Autodesk Fusion 360 part; units mm, degrees
(part 2 of 2)
  arc A37 (11.8839, 4.6211) -> (11.6708, 5.1356) centre (0, 0) ccw
  spline S74 degree 3 poles (11.6708, 5.1356) (11.1523, 5.1719) (10.7664, 5.1326) (10.5094, 5.0835) knots 0 0 0 0 1 1 1 1
  spline S75 degree 3 poles (10.5094, 5.0835) (10.2945, 5.0423) (10.1746, 4.996) (10.1353, 4.9792) knots 0 0 0 0 1 1 1 1
  line L38 (10.1353, 4.9792) -> (9.929, 4.8779)
  arc A38 (9.929, 4.8779) -> (9.5721, 5.5457) centre (0, 0) ccw
  line L39 (9.5721, 5.5457) -> (9.771, 5.6609)
  spline S76 degree 3 poles (9.771, 5.6609) (9.8067, 5.6842) (9.9118, 5.7583) (10.0655, 5.914) knots 0 0 0 0 1 1 1 1
  spline S77 degree 3 poles (10.0655, 5.914) (10.2491, 6.1004) (10.4962, 6.3994) (10.754, 6.8508) knots 0 0 0 0 1 1 1 1
  arc A39 (10.754, 6.8508) -> (10.4447, 7.3137) centre (0, 0) ccw
  spline S78 degree 3 poles (10.4447, 7.3137) (9.929, 7.2483) (9.5582, 7.1344) (9.3157, 7.0361) knots 0 0 0 0 1 1 1 1
  spline S79 degree 3 poles (9.3157, 7.0361) (9.113, 6.9538) (9.0044, 6.8849) (8.9692, 6.8609) knots 0 0 0 0 1 1 1 1
  line L40 (8.9692, 6.8609) -> (8.7866, 6.7212)
  arc A40 (8.7866, 6.7212) -> (8.3062, 7.3065) centre (0, 0) ccw
  line L41 (8.3062, 7.3065) -> (8.4788, 7.4584)
  spline S80 degree 3 poles (8.4788, 7.4584) (8.5093, 7.4882) (8.598, 7.5813) (8.7184, 7.7641) knots 0 0 0 0 1 1 1 1
  spline S81 degree 3 poles (8.7184, 7.7641) (8.862, 7.9827) (9.046, 8.3242) (9.2109, 8.8171) knots 0 0 0 0 1 1 1 1
  arc A41 (9.2109, 8.8171) -> (8.8171, 9.2109) centre (0, 0) ccw
  spline S82 degree 3 poles (8.8171, 9.2109) (8.3242, 9.046) (7.9827, 8.862) (7.7641, 8.7184) knots 0 0 0 0 1 1 1 1
  spline S83 degree 3 poles (7.7641, 8.7184) (7.5813, 8.598) (7.4882, 8.5093) (7.4584, 8.4788) knots 0 0 0 0 1 1 1 1
  line L42 (7.4584, 8.4788) -> (7.3065, 8.3062)
  arc A42 (7.3065, 8.3062) -> (6.7212, 8.7866) centre (0, 0) ccw
  line L43 (6.7212, 8.7866) -> (6.8609, 8.9692)
  spline S84 degree 3 poles (6.8609, 8.9692) (6.8849, 9.0044) (6.9538, 9.113) (7.0361, 9.3157) knots 0 0 0 0 1 1 1 1
  spline S85 degree 3 poles (7.0361, 9.3157) (7.1344, 9.5582) (7.2483, 9.929) (7.3137, 10.4447) knots 0 0 0 0 1 1 1 1
  arc A43 (7.3137, 10.4447) -> (6.8508, 10.754) centre (0, 0) ccw
  spline S86 degree 3 poles (6.8508, 10.754) (6.3994, 10.4962) (6.1004, 10.2491) (5.914, 10.0655) knots 0 0 0 0 1 1 1 1
  spline S87 degree 3 poles (5.914, 10.0655) (5.7583, 9.9118) (5.6842, 9.8067) (5.6609, 9.771) knots 0 0 0 0 1 1 1 1
  line L44 (5.6609, 9.771) -> (5.5457, 9.5721)
  arc A44 (5.5457, 9.5721) -> (4.8779, 9.929) centre (0, 0) ccw
  line L45 (4.8779, 9.929) -> (4.9792, 10.1353)
  spline S88 degree 3 poles (4.9792, 10.1353) (4.996, 10.1746) (5.0423, 10.2945) (5.0835, 10.5094) knots 0 0 0 0 1 1 1 1
  spline S89 degree 3 poles (5.0835, 10.5094) (5.1326, 10.7664) (5.1719, 11.1523) (5.1356, 11.6708) knots 0 0 0 0 1 1 1 1
  arc A45 (5.1356, 11.6708) -> (4.6211, 11.8839) centre (0, 0) ccw
  spline S90 degree 3 poles (4.6211, 11.8839) (4.2287, 11.543) (3.9837, 11.2423) (3.8367, 11.0259) knots 0 0 0 0 1 1 1 1
  spline S91 degree 3 poles (3.8367, 11.0259) (3.7139, 10.8448) (3.6618, 10.7272) (3.6459, 10.6876) knots 0 0 0 0 1 1 1 1
  line L46 (3.6459, 10.6876) -> (3.5717, 10.47)
  arc A46 (3.5717, 10.47) -> (2.8471, 10.6899) centre (0, 0) ccw
  line L47 (2.8471, 10.6899) -> (2.9063, 10.912)
  spline S92 degree 3 poles (2.9063, 10.912) (2.915, 10.9537) (2.937, 11.0804) (2.9356, 11.2992) knots 0 0 0 0 1 1 1 1
  spline S93 degree 3 poles (2.9356, 11.2992) (2.9336, 11.5608) (2.8969, 11.947) (2.76, 12.4485) knots 0 0 0 0 1 1 1 1
  arc A47 (2.76, 12.4485) -> (2.2139, 12.5571) centre (0, 0) ccw
  spline S94 degree 3 poles (2.2139, 12.5571) (1.8956, 12.1462) (1.7139, 11.8034) (1.6119, 11.5625) knots 0 0 0 0 1 1 1 1
  spline S95 degree 3 poles (1.6119, 11.5625) (1.5268, 11.3609) (1.4987, 11.2354) (1.4908, 11.1935) knots 0 0 0 0 1 1 1 1
  line L48 (1.4908, 11.1935) -> (1.4605, 10.9657)
  arc A48 (1.4605, 10.9657) -> (0.7069, 11.0399) centre (0, 0) ccw
  line L49 (0.7069, 11.0399) -> (0.7216, 11.2693)
  spline S96 degree 3 poles (0.7216, 11.2693) (0.7221, 11.3119) (0.7189, 11.4405) (0.6748, 11.6548) knots 0 0 0 0 1 1 1 1
  spline S97 degree 3 poles (0.6748, 11.6548) (0.6218, 11.911) (0.5105, 12.2826) (0.2784, 12.7477) knots 0 0 0 0 1 1 1 1
  arc A49 (0.2784, 12.7477) -> (-0.2784, 12.7477) centre (0, 0) ccw
  spline S98 degree 3 poles (-0.2784, 12.7477) (-0.5105, 12.2826) (-0.6218, 11.911) (-0.6748, 11.6548) knots 0 0 0 0 1 1 1 1
  spline S99 degree 3 poles (-0.6748, 11.6548) (-0.7189, 11.4405) (-0.7221, 11.3119) (-0.7216, 11.2693) knots 0 0 0 0 1 1 1 1
  line L50 (-0.7216, 11.2693) -> (-0.7069, 11.0399)
  arc A50 (-0.7069, 11.0399) -> (-1.4605, 10.9657) centre (0, 0) ccw
  line L51 (-1.4605, 10.9657) -> (-1.4908, 11.1935)
  spline S100 degree 3 poles (-1.4908, 11.1935) (-1.4987, 11.2354) (-1.5268, 11.3609) (-1.6119, 11.5625) knots 0 0 0 0 1 1 1 1
  spline S101 degree 3 poles (-1.6119, 11.5625) (-1.7139, 11.8034) (-1.8956, 12.1462) (-2.2139, 12.5571) knots 0 0 0 0 1 1 1 1
  arc A51 (-2.2139, 12.5571) -> (-2.76, 12.4485) centre (0, 0) ccw
  spline S102 degree 3 poles (-2.76, 12.4485) (-2.8969, 11.947) (-2.9336, 11.5608) (-2.9356, 11.2992) knots 0 0 0 0 1 1 1 1
  spline S103 degree 3 poles (-2.9356, 11.2992) (-2.937, 11.0804) (-2.915, 10.9537) (-2.9063, 10.912) knots 0 0 0 0 1 1 1 1
  line L52 (-2.9063, 10.912) -> (-2.8471, 10.6899)
  arc A52 (-2.8471, 10.6899) -> (-3.5717, 10.47) centre (0, 0) ccw
  line L53 (-3.5717, 10.47) -> (-3.6459, 10.6876)
  spline S104 degree 3 poles (-3.6459, 10.6876) (-3.6618, 10.7272) (-3.7139, 10.8448) (-3.8367, 11.0259) knots 0 0 0 0 1 1 1 1
  spline S105 degree 3 poles (-3.8367, 11.0259) (-3.9837, 11.2423) (-4.2287, 11.543) (-4.6211, 11.8839) knots 0 0 0 0 1 1 1 1
  arc A53 (-4.6211, 11.8839) -> (-5.1356, 11.6708) centre (0, 0) ccw
  spline S106 degree 3 poles (-5.1356, 11.6708) (-5.1719, 11.1523) (-5.1326, 10.7664) (-5.0835, 10.5094) knots 0 0 0 0 1 1 1 1
  spline S107 degree 3 poles (-5.0835, 10.5094) (-5.0423, 10.2945) (-4.996, 10.1746) (-4.9792, 10.1353) knots 0 0 0 0 1 1 1 1
  line L54 (-4.9792, 10.1353) -> (-4.8779, 9.929)
  arc A54 (-4.8779, 9.929) -> (-5.5457, 9.5721) centre (0, 0) ccw
  line L55 (-5.5457, 9.5721) -> (-5.6609, 9.771)
  spline S108 degree 3 poles (-5.6609, 9.771) (-5.6842, 9.8067) (-5.7583, 9.9118) (-5.914, 10.0655) knots 0 0 0 0 1 1 1 1
  spline S109 degree 3 poles (-5.914, 10.0655) (-6.1004, 10.2491) (-6.3994, 10.4962) (-6.8508, 10.754) knots 0 0 0 0 1 1 1 1
  arc A55 (-6.8508, 10.754) -> (-7.3137, 10.4447) centre (0, 0) ccw
  spline S110 degree 3 poles (-7.3137, 10.4447) (-7.2483, 9.929) (-7.1344, 9.5582) (-7.0361, 9.3157) knots 0 0 0 0 1 1 1 1
  spline S111 degree 3 poles (-7.0361, 9.3157) (-6.9538, 9.113) (-6.8849, 9.0044) (-6.8609, 8.9692) knots 0 0 0 0 1 1 1 1
  line L56 (-6.8609, 8.9692) -> (-6.7212, 8.7866)
  arc A56 (-6.7212, 8.7866) -> (-7.3065, 8.3062) centre (0, 0) ccw
  line L57 (-7.3065, 8.3062) -> (-7.4584, 8.4788)
  spline S112 degree 3 poles (-7.4584, 8.4788) (-7.4882, 8.5093) (-7.5813, 8.598) (-7.7641, 8.7184) knots 0 0 0 0 1 1 1 1
  spline S113 degree 3 poles (-7.7641, 8.7184) (-7.9827, 8.862) (-8.3242, 9.046) (-8.8171, 9.2109) knots 0 0 0 0 1 1 1 1
  arc A57 (-8.8171, 9.2109) -> (-9.2109, 8.8171) centre (0, 0) ccw
  spline S114 degree 3 poles (-9.2109, 8.8171) (-9.046, 8.3242) (-8.862, 7.9827) (-8.7184, 7.7641) knots 0 0 0 0 1 1 1 1
  spline S115 degree 3 poles (-8.7184, 7.7641) (-8.598, 7.5813) (-8.5093, 7.4882) (-8.4788, 7.4584) knots 0 0 0 0 1 1 1 1
  line L58 (-8.4788, 7.4584) -> (-8.3062, 7.3065)
  arc A58 (-8.3062, 7.3065) -> (-8.7866, 6.7212) centre (0, 0) ccw
  line L59 (-8.7866, 6.7212) -> (-8.9692, 6.8609)
  spline S116 degree 3 poles (-8.9692, 6.8609) (-9.0044, 6.8849) (-9.113, 6.9538) (-9.3157, 7.0361) knots 0 0 0 0 1 1 1 1
  spline S117 degree 3 poles (-9.3157, 7.0361) (-9.5582, 7.1344) (-9.929, 7.2483) (-10.4447, 7.3137) knots 0 0 0 0 1 1 1 1
  arc A59 (-10.4447, 7.3137) -> (-10.754, 6.8508) centre (0, 0) ccw
  spline S118 degree 3 poles (-10.754, 6.8508) (-10.4962, 6.3994) (-10.2491, 6.1004) (-10.0655, 5.914) knots 0 0 0 0 1 1 1 1
  spline S119 degree 3 poles (-10.0655, 5.914) (-9.9118, 5.7583) (-9.8067, 5.6842) (-9.771, 5.6609) knots 0 0 0 0 1 1 1 1
  line L60 (-9.771, 5.6609) -> (-9.5721, 5.5457)
  arc A60 (-9.5721, 5.5457) -> (-9.929, 4.8779) centre (0, 0) ccw
  line L61 (-9.929, 4.8779) -> (-10.1353, 4.9792)
  spline S120 degree 3 poles (-10.1353, 4.9792) (-10.1746, 4.996) (-10.2945, 5.0423) (-10.5094, 5.0835) knots 0 0 0 0 1 1 1 1
  spline S121 degree 3 poles (-10.5094, 5.0835) (-10.7664, 5.1326) (-11.1523, 5.1719) (-11.6708, 5.1356) knots 0 0 0 0 1 1 1 1
  arc A61 (-11.6708, 5.1356) -> (-11.8839, 4.6211) centre (0, 0) ccw
  spline S122 degree 3 poles (-11.8839, 4.6211) (-11.543, 4.2287) (-11.2423, 3.9837) (-11.0259, 3.8367) knots 0 0 0 0 1 1 1 1
  spline S123 degree 3 poles (-11.0259, 3.8367) (-10.8448, 3.7139) (-10.7272, 3.6618) (-10.6876, 3.6459) knots 0 0 0 0 1 1 1 1
  line L62 (-10.6876, 3.6459) -> (-10.47, 3.5717)
  arc A62 (-10.47, 3.5717) -> (-10.6899, 2.8471) centre (0, 0) ccw
  line L63 (-10.6899, 2.8471) -> (-10.912, 2.9063)
  spline S124 degree 3 poles (-10.912, 2.9063) (-10.9537, 2.915) (-11.0804, 2.937) (-11.2992, 2.9356) knots 0 0 0 0 1 1 1 1
  spline S125 degree 3 poles (-11.2992, 2.9356) (-11.5608, 2.9336) (-11.947, 2.8969) (-12.4485, 2.76) knots 0 0 0 0 1 1 1 1
  arc A63 (-12.4485, 2.76) -> (-12.5571, 2.2139) centre (0, 0) ccw
  spline S126 degree 3 poles (-12.5571, 2.2139) (-12.1462, 1.8956) (-11.8034, 1.7139) (-11.5625, 1.6119) knots 0 0 0 0 1 1 1 1
  spline S127 degree 3 poles (-11.5625, 1.6119) (-11.3609, 1.5268) (-11.2354, 1.4987) (-11.1935, 1.4908) knots 0 0 0 0 1 1 1 1
  circle A64 centre (0, 0) radius 4
  dimension "d3" = 8
  constraint concentric A4 A64
  measures "d3" diameter of A64
extrude "Extrude2" add sketch "Sketch1 (2)" against normal blind 25 contours A64 in component "Spur Gear (32 teeth)"
extrude "Extrude3" add sketch "Sketch1 (2)" against normal blind 40 contours A64 in component "Spur Gear (32 teeth)"
extrude "Extrude4" add sketch "Sketch1 (2)" along normal blind 15 contours A64 in component "Spur Gear (32 teeth)"
sketch "Sketch2 (2)" plane through (0, 40, 0) normal (0, 1, 0) x (-1, 0, 0)
  circle A0 centre (0, 0) radius 4
extrude "Extrude5" cut sketch "Sketch2 (2)" against normal blind 1 in component "Spur Gear (32 teeth)"
sketch "Sketch3" plane through (0, 39, 0) normal (0, 1, 0) x (-1, 0, 0)
  circle A0 centre (0, 0) radius 4
  circle A1 centre (0, 0) radius 2
  dimension "d13" = 4
  constraint concentric A0 A1
  measures "d13" diameter of A1
extrude "Extrude6" cut sketch "Sketch3" against normal blind 5 contours A1 in component "Spur Gear (32 teeth)"
extrude "Extrude7" add 1 faces at (-3.311, 39, -0.2981) along direction (0, 1, 0) blind 1 in component "Spur Gear (32 teeth)"
extrude "Extrude8" cut 1 faces at (1.2456, -15, 0.0132) along direction (0, 1, 0) blind 1 in component "Spur Gear (32 teeth)"
thread "Thread1" "ISO Metric profile 4.0 M4x0.7 6H" major diameter 4.1095 minor diameter 3.332 pitch 0.7 angle 60 modelled right hand crest width 0.193 on face at (-1.9975, 38, -0.0997) crest through (-1.666, 39.825, 0) in component "Spur Gear (32 teeth)"
sketch "Sketch4" plane through (0, 40, 0) normal (0, 1, 0) x (-1, 0, 0)
  circle A0 centre (0, 0) radius 4
  circle A1 centre (0, 0) radius 2.5
  dimension "d22" = 5
  measures "d22" diameter of A1
extrude "Extrude10" cut sketch "Sketch4" against normal blind 6 contours A1 in component "Spur Gear (32 teeth)"
extrude "Extrude11" add 1 faces at (-0.4919, 34, 0.773) along direction (0, 1, 0) blind 6 in component "Spur Gear (32 teeth)"
extrude "Extrude12" cut 1 faces at (1.2456, 40, 0.0132) along direction (0, -1, 0) blind 15 in component "Spur Gear (32 teeth)"
extrude "Extrude13" cut 1 faces at (1.2456, -14, 0.0132) along direction (0, 1, 0) blind 14 in component "Spur Gear (32 teeth)"
extrude "Extrude14" cut sketch "Sketch1 (2)" against normal blind 50 contours A64 in component "Spur Gear (32 teeth)"
extrude "Extrude15" cut 1 faces at (-8.6933, 25, 0) along direction (0, -1, 0) blind 10.55 in component "Spur Gear (32 teeth)"
component "Spur Gear (32 teeth)" placed x (1, 0, 0) y (0, 1, 0) z (0, 0, 1) at (0, 0, 0)
